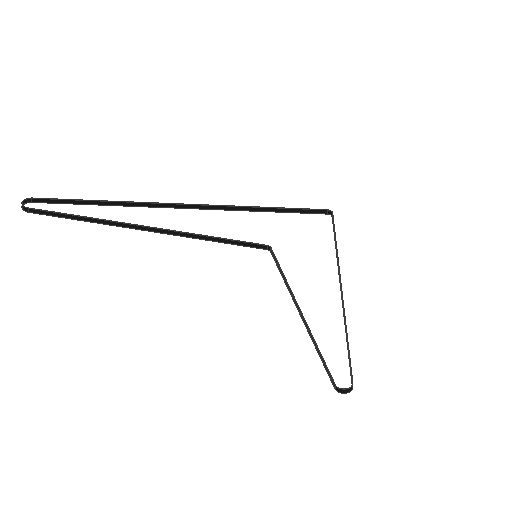
# Autodesk Inventor part: COTS_GENERIC_Z_Axis_GT2_Timing_Belt
Saved by Autodesk Inventor 2026.1 (Build 301233000, 233)
## iProperties
Created: 2016-06-25
Part Number: COTS_GENERIC_Z_Axis_GT2_Timing_Belt
Material: Ogólny
Document SubType Name: Modeling
Designer: Andrzej
Density: 1 g/cm^3
Appearance: Kauczuk - czarny
Mass: 5.00021 g
Surface Area: 171.038 cm^2
Volume: 5.00021 cm^3
Author: Andrzej
Autodesk Inventor part; units mm, degrees
ref_plane "YZ Plane" through (0, 0, 0) normal (1, 0, 0) x (0, 1, 0)
ref_plane "XZ Plane" through (0, 0, 0) normal (0, 1, 0) x (-1, 0, 0)
ref_plane "XY Plane" through (0, 0, 0) normal (0, 0, 1) x (1, 0, 0)
sketch "Szkic1" plane through (0, 0, 0) normal (0, 0, 1) x (1, 0, 0)
  arc A0 (11.9269, 375.7404) -> (3.9766, 375.7404) centre (7.9517, 371.1796) ccw
  arc A1 (-263.2304, 142.8463) -> (-251.4901, 126.3567) centre (-256.5483, 135.1796) ccw
  arc A2 (267.3935, 126.3567) -> (279.1339, 142.8463) centre (272.4517, 135.1796) ccw
  arc A3 (10.9359, 273.3848) -> (4.9676, 273.3848) centre (7.9517, 268.1796) ccw
  line L0 (-251.4901, 126.3567) -> (4.9676, 273.3848)
  line L1 (10.9359, 273.3848) -> (267.3935, 126.3567)
  line L2 (-263.2304, 142.8463) -> (3.9766, 375.7404)
  line L3 (11.9269, 375.7404) -> (279.1339, 142.8463)
  arc A4 (12.3539, 376.2304) -> (3.5495, 376.2304) centre (7.9517, 371.1796) ccw
  line L4 (12.3539, 376.2304) -> (279.561, 143.3363)
  arc A5 (267.0703, 125.7928) -> (279.561, 143.3363) centre (272.4517, 135.1796) ccw
  line L5 (267.0703, 125.7928) -> (10.6126, 272.8209)
  arc A6 (10.6126, 272.8209) -> (5.2908, 272.8209) centre (7.9517, 268.1796) ccw
  line L6 (5.2908, 272.8209) -> (-251.1668, 125.7928)
  arc A7 (-263.6575, 143.3363) -> (-251.1668, 125.7928) centre (-256.5483, 135.1796) ccw
  line L7 (-263.6575, 143.3363) -> (3.5495, 376.2304)
  point P0 (0, 0)
  dimension "d0" = 264.5
  dimension "d1" = 264.5
  dimension "d2" = 236
  dimension "d3" = 236
  dimension "d10" = 0
  dimension "d11" = 103
  dimension "d16" = 12.1
  dimension "d17" = 20.34
  dimension "d18" = 20.34
  dimension "d19" = 12
  dimension "d20" = 0.65
  constraints: 16 end point, 16 point on circle, 8 centre point, 8 tangent, 4 coincident, 7 other
  measures "d0" horizontal distance of point (7.952, 371.18) point (-256.548, 135.18)
  measures "d1" horizontal distance of point (272.452, 135.18) point (7.952, 371.18)
  measures "d2" vertical distance of point (-256.548, 135.18) point (7.952, 371.18)
  measures "d3" vertical distance of point (272.452, 135.18) point (7.952, 371.18)
  measures "d10" horizontal distance of point (7.952, 268.18) point (7.952, 371.18)
  measures "d11" distance of point (7.952, 268.18) point (7.952, 371.18)
  measures "d16" diameter of A0
  measures "d17" diameter of A1
  measures "d18" diameter of A2
  measures "d19" diameter of A3
  measures "d20" distance between parallel lines of L2 L7
extrude "Wyciągnięcie proste2" add sketch "Szkic1" along normal blind 6
equation "\"d1\" = d0"
equation "\"d3\" = d2"
